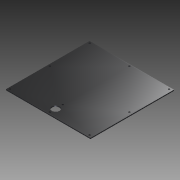
# Autodesk Inventor part: EnclosurePanelRight
Saved by Autodesk Inventor 2015 SP1 (Build 190203100, 203)
## iProperties
Category: Panel
Created: 2015-01-12
Part Number: EnclosurePanelRight
Material: ABS Plastic
Document SubType Name: Modeling
Designer: Jack
Density: 1.06 g/cm^3
Appearance: Smooth - Dark Gray
Mass: 595.148 g
Surface Area: 2867.62 cm^2
Volume: 561.46 cm^3
Vendor: Tap Plastics
Catalog Web Link: N/A
Author: Jack
Title: Enclosure Panel Right
Autodesk Inventor part; units mm, degrees
ref_plane "YZ Plane" through (0, 0, 0) normal (1, 0, 0) x (0, 1, 0)
ref_plane "XZ Plane" through (0, 0, 0) normal (0, 1, 0) x (-1, 0, 0)
ref_plane "XY Plane" through (0, 0, 0) normal (0, 0, 1) x (1, 0, 0)
sketch "Sketch1" plane through (0, 0, 0) normal (0, 0, 1) x (1, 0, 0)
  line L0 (0, 0) -> (424.7625, 0)
  line L1 (424.7625, 0) -> (424.7625, 420)
  line L2 (424.7625, 420) -> (0, 420)
  line L3 (0, 420) -> (0, 0)
  dimension "d0" = 424.7625
  dimension "d1" = 420
  constraints: 8 end point, 2 parallel, 1 horizontal, 1 perpendicular
  measures "d0" distance of L2.end L1.end
  measures "d1" distance of L0.end L1.end
extrude "Extrusion1" add sketch "Sketch1" along normal blind 4.7625
sketch "Sketch3" plane through (0, 0, 4.7625) normal (0, 0, 1) x (1, 0, 0)
  line L0 (0, 0) -> (424.7625, 0) projected
  line L1 (0, 420) -> (0, 0) projected
  circle A0 centre (209.8815, 40) radius 19.05
  dimension "d13" = 38.1
  dimension "d14" = 209.8815
  dimension "d30" = 40
  constraints: 1 centre point
  measures "d13" diameter of A0
  measures "d14" distance from line of L1 A0.centre
  measures "d30" distance from line of L0 A0.centre
extrude "Extrusion2" cut sketch "Sketch3" against normal up to next
sketch "Sketch5" plane through (0, 0, 4.7625) normal (0, 0, 1) x (1, 0, 0)
  circle A0 centre (209.8815, 40) radius 19.05 projected
  point P0 (193.8815, 56)
  point P1 (225.8815, 56)
  point P2 (193.8815, 24)
  point P3 (225.8815, 24)
  dimension "d31" = 32
  dimension "d32" = 32
  dimension "d33" = 16
  dimension "d34" = 16
  constraints: 2 horizontal alignment, 2 vertical alignment
  measures "d31" distance of point (225.881, 56) point (225.881, 24)
  measures "d32" distance of point (225.881, 56) point (193.881, 56)
  measures "d33" horizontal distance of A0.centre point (193.881, 56)
  measures "d34" horizontal distance of A0.centre point (225.881, 56)
hole "Hole2" at (193.8815, 56, 4.7625) at (225.8815, 56, 4.7625) at (193.8815, 24, 4.7625) at (225.8815, 24, 4.7625) direction (0, 0, -1) diameter 3.5 end through all
sketch "Sketch6" plane through (0, 0, 4.7625) normal (0, 0, 1) x (1, 0, 0)
  line L0 (0, 0) -> (424.7625, 0) projected
  line L1 (424.7625, 0) -> (424.7625, 420) projected
  line L2 (424.7625, 420) -> (0, 420) projected
  line L3 (0, 420) -> (0, 0) projected
  circle A0 centre (10, 410) radius 2.25
  circle A1 centre (410, 410) radius 2.25
  circle A2 centre (10, 10) radius 2.25
  circle A3 centre (410, 10) radius 2.25
  circle A4 centre (10, 210) radius 2.25
  circle A5 centre (410, 210) radius 2.25
  circle A6 centre (209.8815, 410) radius 2.25
  circle A7 centre (209.8815, 10) radius 2.25
  circle A8 centre (209.8815, 75) radius 2.25
  dimension "d42" = 4.5
  dimension "d43" = 10
  dimension "d44" = 10
  dimension "d45" = 14.7625
  dimension "d46" = 10
  dimension "d47" = 10
  dimension "d48" = 210
  dimension "d51" = 209.8815
  dimension "d55" = 75
  constraints: 9 centre point, 8 equal radius, 6 vertical alignment, 4 horizontal alignment
  measures "d42" diameter of A0
  measures "d43" distance from line of L2 A0.centre
  measures "d44" distance from line of L3 A0.centre
  measures "d45" distance from line of L1 A1.centre
  measures "d46" distance from line of L2 A1.centre
  measures "d47" distance from line of L0 A2.centre
  measures "d48" distance from line of L0 A5.centre
  measures "d51" distance from line of L3 A6.centre
  measures "d55" distance from line of L0 A8.centre
extrude "Extrusion3" cut sketch "Sketch6" against normal up to next contours A0 | A1 | A2 | A3 | A4 | A5 | A6 | A7 | A8
chamfer "Chamfer1" distance 2 angle 45 9 edges at (7.75, 410, 4.7625) (207.6315, 410, 4.7625) (407.75, 410, 4.7625) (407.75, 210, 4.7625) (7.75, 210, 4.7625) (7.75, 10, 4.7625) (207.6315, 10, 4.7625) (407.75, 10, 4.7625) (207.6315, 75, 4.7625)
body "Solid1"
